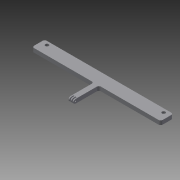
# Autodesk Inventor part: WebcamBase
Saved by Autodesk Inventor 2015 (Build 190159000, 159)
## iProperties
Created: 2015-05-12
Part Number: WebcamBase
Material: Generic
Document SubType Name: Modeling
Designer: Kurtis
Density: 1 g/cm^3
Appearance: Default
Author: Kurtis
Autodesk Inventor part; units mm, degrees
ref_plane "YZ Plane" through (0, 0, 0) normal (1, 0, 0) x (0, 1, 0)
ref_plane "XZ Plane" through (0, 0, 0) normal (0, 1, 0) x (-1, 0, 0)
ref_plane "XY Plane" through (0, 0, 0) normal (0, 0, 1) x (1, 0, 0)
sketch "Sketch1" plane through (0, 0, 0) normal (0, 0, 1) x (1, 0, 0)
  line L0 (254, 0) -> (254, 25)
  line L1 (254, 25) -> (0, 25)
  line L2 (0, 25) -> (0, 0)
  line L3 (0, 25) -> (0, 21) construction
  line L4 (0, 21) -> (8.5, 21) construction
  line L5 (8.5, 21) -> (11.75, 21) construction
  line L6 (11.75, 21) -> (11.75, 17.75) construction
  circle A0 centre (11.75, 17.75) radius 3.25
  line L7 (254, 25) -> (254, 21) construction
  line L8 (254, 21) -> (245.5, 21) construction
  line L9 (245.5, 21) -> (245.5, 17.75) construction
  line L10 (245.5, 17.75) -> (242.25, 17.75) construction
  circle A1 centre (242.25, 17.75) radius 3.25
  line L11 (132, -50) -> (132, 0)
  line L12 (122, -50) -> (122, 0)
  line L13 (0, 0) -> (122, 0)
  line L14 (132, 0) -> (254, 0)
  line L15 (122, -50) -> (124, -50)
  line L16 (124, -50) -> (124, -42)
  line L17 (124, -42) -> (126, -42)
  line L18 (126, -42) -> (126, -50)
  line L19 (126, -50) -> (128, -50)
  line L20 (128, -50) -> (128, -42)
  line L21 (128, -42) -> (130, -42)
  line L22 (130, -42) -> (130, -50)
  line L23 (130, -50) -> (132, -50)
  dimension "d0" = 254
  dimension "d1" = 25
  dimension "d2" = 4
  dimension "d3" = 8.5
  dimension "d4" = 3.25
  dimension "d5" = 3.25
  dimension "d6" = 4
  dimension "d7" = 8.5
  dimension "d8" = 3.25
  dimension "d9" = 3.25
  dimension "d13" = 122
  dimension "d14" = 242.25
  dimension "d16" = 2
  dimension "d17" = 8
  dimension "d18" = 2
  dimension "d19" = 8
  dimension "d20" = 2
  dimension "d21" = 8
  dimension "d22" = 2
  dimension "d23" = 124
  dimension "d24" = 63
  constraints: 48 end point, 14 perpendicular, 8 point on line, 5 horizontal, 2 coincident, 1 horizontal alignment, 1 parallel, 1 vertical, 1 vertical alignment, 4 other
  measures "d0" distance of L2.end L0.start
  measures "d1" distance of L0.start L0.end
  measures "d2" distance of L1.end L3.end
  measures "d3" distance of L3.end L4.end
  measures "d4" distance of L4.end L5.end
  measures "d5" distance of L5.end L6.end
  measures "d6" distance of L0.end L7.end
  measures "d7" distance of L7.end L8.end
  measures "d8" distance of L8.end L9.end
  measures "d9" distance of L9.end L10.end
  measures "d13" distance between parallel lines of L11 L0
  measures "d14" distance between parallel lines of L6 L0
  measures "d16" distance of L12.start L15.end
  measures "d17" distance of L15.end L16.end
  measures "d18" distance of L16.end L17.end
  measures "d19" distance of L17.end L18.end
  measures "d20" distance of L18.end L19.end
  measures "d21" distance of L19.end L20.end
  measures "d22" distance of L20.end L21.end
  measures "d23" distance between parallel lines of L22 L0
  measures "d24" distance between parallel lines of L21 L8
extrude "Extrusion1" add sketch "Sketch1" along normal blind 8
sketch "Sketch3" plane through (132, -50, 0) normal (1, 0, 0) x (0, 0, -1)
  line L0 (0, 0) -> (-8, 0) projected
  line L1 (0, 8) -> (-8, 8) projected
  line L2 (0, 0) -> (-8, 0) construction
  line L3 (-4, 0) -> (-4, 8) construction
  circle A0 centre (-4, 4) radius 1
  point P0 (0, 50)
  point P1 (-12, 0)
  point P2 (-12, 8)
  dimension "d39" = 2
  constraints: 3 midpoint, 2 end point, 1 centre point
  measures "d39" diameter of A0
extrude "Extrusion3" cut sketch "Sketch3" against normal blind 46.75
fillet "Fillet2" radius 4 6 edges at (127, -50, 8) (127, -50, 0) (123, -50, 0) (123, -50, 8) (131, -50, 0) (131, -50, 8)
fillet "Fillet4" radius 4 6 edges at (0, 25, 4) (0, 0, 4) (122, 0, 4) (132, 0, 4) (254, 0, 4) (254, 25, 4)
body "Solid1"
